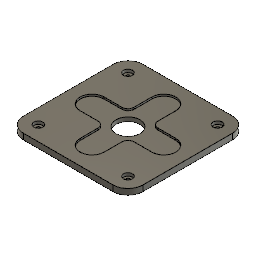
Entrega_MecanizadoMTO8 (Autodesk Fusion 360 design; units mm, degrees)
Autodesk Fusion 360 part; units mm, degrees
sketch "Boceto1" plane through (0, 0, 0) normal (0, 1, 0) x (1, 0, 0)
  line L0 (-75, 100) -> (75, 100)
  line L1 (100, 75) -> (100, -75)
  line L2 (75, -100) -> (-75, -100)
  line L3 (-100, -75) -> (-100, 75)
  line L4 (-100, 100) -> (100, -100) construction
  line L5 (100, 100) -> (-100, -100) construction
  arc A0 (-75, 100) -> (-100, 75) centre (-75, 75) ccw
  arc A1 (-100, -75) -> (-75, -100) centre (-75, -75) ccw
  arc A2 (75, -100) -> (100, -75) centre (75, -75) ccw
  arc A3 (100, 75) -> (75, 100) centre (75, 75) ccw
  circle A4 centre (-75, 75) radius 3
  circle A5 centre (75, 75) radius 3
  circle A6 centre (-75, -75) radius 3
  circle A7 centre (75, -75) radius 3
  circle A8 centre (-75, 75) radius 7.5
  circle A9 centre (75, 75) radius 7.5
  circle A10 centre (-75, -75) radius 7.5
  circle A11 centre (75, -75) radius 7.5
  line L6 (0, 0) -> (0, 60)
  line L7 (20, 0) -> (20, 60)
  line L8 (-20, 0) -> (-20, 60)
  line L9 (0, -20) -> (-60, -20)
  line L10 (0, 0) -> (-60, 0)
  line L11 (0, 20) -> (-60, 20)
  line L12 (20, 0) -> (20, -60)
  line L13 (0, 0) -> (0, -60)
  line L14 (-20, 0) -> (-20, -60)
  line L15 (0, 20) -> (60, 20)
  line L16 (0, 0) -> (60, 0)
  line L17 (0, -20) -> (60, -20)
  arc A12 (20, 60) -> (-20, 60) centre (0, 60) ccw
  arc A13 (-60, 20) -> (-60, -20) centre (-60, 0) ccw
  arc A14 (-20, -60) -> (20, -60) centre (0, -60) ccw
  arc A15 (60, -20) -> (60, 20) centre (60, 0) ccw
  circle A16 centre (0, 0) radius 20
  dimension "d1" = 200
  dimension "d2" = 200
  dimension "d3" = 25
  dimension "d4" = 6
  dimension "d5" = 6
  dimension "d6" = 6
  dimension "d7" = 6
  dimension "d8" = 15
  dimension "d9" = 15
  dimension "d10" = 15
  dimension "d11" = 15
  dimension "d12" = 60
  dimension "d13" = 20
  dimension "d14" = -20
  dimension "d16" = 360
  dimension "d18" = 360
  dimension "d25" = 40
  constraint horizontal L0
  constraint perpendicular L0 L1
  constraint parallel L0 L2
  constraint parallel L1 L3
  constraint coincident L4 L6.start
  constraint coincident L5 L6.start
  constraint coincident L6.start L10.start
  constraint coincident L4.start L0
  constraint coincident L4.start L3
  constraint tangent L0 A0
  constraint tangent L3 A0
  constraint coincident L5.end L3
  constraint coincident L5.end L2
  constraint tangent L3 A1
  constraint tangent L2 A1
  constraint equal A0 A1
  constraint coincident L4.end L2
  constraint coincident L4.end L1
  constraint tangent L2 A2
  constraint tangent L1 A2
  constraint equal A0 A2
  constraint coincident L5.start L1
  constraint coincident L5.start L0
  constraint tangent L1 A3
  constraint tangent L0 A3
  constraint equal A0 A3
  constraint concentric A0 A4
  constraint concentric A3 A5
  constraint concentric A1 A6
  constraint concentric A2 A7
  constraint concentric A4 A8
  constraint concentric A3 A9
  constraint concentric A1 A10
  constraint concentric A7 A11
  constraint vertical L6
  constraint tangent L7 A12
  constraint tangent L8 A12
  measures "d1" distance of L4.end L5.end
  measures "d2" distance of L5.start L4.end
  measures "d3" radius of A0
  measures "d4" diameter of A4
  measures "d5" diameter of A5 L0.start
  measures "d6" diameter of A6
  measures "d7" diameter of A7
  measures "d8" diameter of A8
  measures "d9" diameter of A9 L0.start
  measures "d10" diameter of A10
  measures "d11" diameter of A11
  measures "d12" distance of L6.start L6.end
  measures "d25" diameter of A16
extrude "Extruir1" add sketch "Boceto1" along normal blind 10 contours L0 L1 L2 L3 A0 A1 A2 A3
extrude "Extruir2" add sketch "Boceto1" along normal blind 7 contours L6 L10 A16 | L10 L13 A16 | L13 L16 A16 | L6 L16 A16 | L8 L11 A16 | L7 L8 L11 L15 A12 | L7 L15 A16 | L8 L9 L11 L14 A13 | L9 L14 A16 | L9 L12 L14 L17 A14 | L12 L17 A16 | L7 L12 L15 L17 A15
extrude "Extruir3" add sketch "Boceto1" along normal blind 5 contours A8 | A9 | A10 | A11
extrude "Extruir4" cut sketch "Boceto1" along normal blind 40 contours L6 L10 A16 | L10 L13 A16 | L13 L16 A16 | L6 L16 A16
fillet "Empalme1" radius 10 4 edges at (-20, 8.5, -20) (20, 8.5, -20) (-20, 8.5, 20) (20, 8.5, 20)
